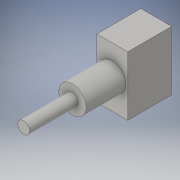
# Autodesk Inventor part: msheehan_switch
Saved by Autodesk Inventor 2016 (Build 200138000, 138)
## iProperties
Created: 2017-08-30
Part Number: msheehan_switch
Material: Generic
Document SubType Name: Modeling
Designer: student
Density: 1 g/cm^3
Appearance: Default
Author: student
Autodesk Inventor part; units mm, degrees
ref_plane "YZ Plane" through (0, 0, 0) normal (1, 0, 0) x (0, 1, 0)
ref_plane "XZ Plane" through (0, 0, 0) normal (0, 1, 0) x (-1, 0, 0)
ref_plane "XY Plane" through (0, 0, 0) normal (0, 0, 1) x (1, 0, 0)
sketch "Sketch2" plane through (0, 0, 0) normal (0, 0, 1) x (1, 0, 0)
  line L0 (0, 0) -> (6.604, 0)
  line L1 (6.604, 0) -> (6.604, 12.7)
  line L2 (6.604, 12.7) -> (0, 12.7)
  line L3 (0, 12.7) -> (0, 0)
  dimension "d0" = 6.604
  dimension "d1" = 12.7
  constraints: 8 end point, 2 parallel, 1 horizontal, 1 perpendicular
  measures "d0" distance of L2.end L1.end
  measures "d1" distance of L1.end L0.end
extrude "Extrusion1" add sketch "Sketch2" along normal blind 9.398
sketch "Sketch3" plane through (0, 0, 9.398) normal (0, 0, 1) x (1, 0, 0)
  line L0 (6.604, 12.7) -> (0, 12.7) projected
  line L1 (3.302, 9.398) -> (3.302, 3.556) construction
  circle A0 centre (3.302, 6.477) radius 2.921
  point P0 (0, 0)
  dimension "d5" = 5.842
  constraints: 2 end point, 1 midpoint, 1 vertical, 1 vertical alignment, 2 other
  measures "d5" distance of L1.start L1.end
extrude "Extrusion2" add sketch "Sketch3" along normal blind 8.509
sketch "Sketch4" plane through (3.302, 6.477, 17.907) normal (0, 0, 1) x (1, 0, 0)
  circle A0 centre (0, 0) radius 1.27
  point P0 (-3.302, -6.477)
  dimension "d8" = 2.54
  constraints: 1 centre point
  measures "d8" diameter of A0
extrude "Extrusion3" add sketch "Sketch4" along normal blind 10.414
body "Solid1"
